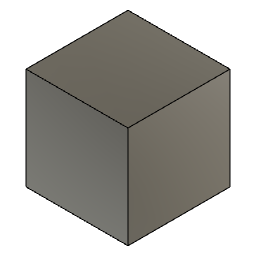
練習用_加藤 (Autodesk Fusion 360 design; units mm, degrees)
Autodesk Fusion 360 part; units mm, degrees
sketch "スケッチ1" plane through (0, 0, 0) normal (0, 0, 1) x (1, 0, 0)
  line L0 (0, 50) -> (50, 50)
  line L1 (50, 50) -> (50, 0)
  line L2 (50, 0) -> (0, 0)
  line L3 (0, 0) -> (0, 50)
  constraint horizontal L0
  constraint vertical L1
  constraint horizontal L2
  constraint vertical L3
extrude "押し出し1" add sketch "スケッチ1" along normal blind 50
